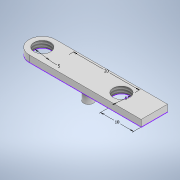
# Autodesk Inventor part: link
Saved by Autodesk Inventor 2021 (Build 250183000, 183)
## iProperties
Created: 2020-11-29
Part Number: link
Material: Generic
Document SubType Name: Modeling
Designer: awitc
Density: 1 g/cm^3
Appearance: Default
Author: awitc
Autodesk Inventor part; units mm, degrees
ref_plane "YZ Plane" through (0, 0, 0) normal (1, 0, 0) x (0, 1, 0)
ref_plane "XZ Plane" through (0, 0, 0) normal (0, 1, 0) x (-1, 0, 0)
ref_plane "XY Plane" through (0, 0, 0) normal (0, 0, 1) x (1, 0, 0)
sketch "Sketch1" plane through (0, 0, 0) normal (0, 1, 0) x (-1, 0, 0)
  line L0 (0, 4) -> (-20, 4)
  line L1 (-20, 4) -> (-20, -4)
  line L2 (-20, -4) -> (0, -4)
  circle A0 centre (-20, 0) radius 4
  circle A1 centre (-20, 0) radius 2.5
  line L3 (-20, -4) -> (-30, -4)
  line L4 (-30, -4) -> (-30, 4)
  line L5 (-30, 4) -> (-20, 4)
  line L6 (-20, 4) -> (-20, -4)
  circle A2 centre (4, 0) radius 4
  circle A3 centre (4, 0) radius 2.5
  line L7 (0, 4) -> (4, 4)
  line L8 (4, -4) -> (0, -4)
  point P0 (-20, -2.5)
  point P1 (-20, 2.5)
  dimension "d32" = 20
  dimension "d34" = 5
  dimension "d47" = 10
  dimension "d48" = 5
  constraints: 18 end point, 4 parallel, 3 centre point, 2 coincident, 2 horizontal, 2 perpendicular, 2 point on circle, 2 tangent, 1 midpoint, 3 other
  measures "d32" distance of L2.end L1.end
  measures "d34" diameter of A1
  measures "d47" distance of L4.end L5.end
  measures "d48" diameter of A3
extrude "Extrusion1" add sketch "Sketch1" along normal blind 2 contours L7 A2 L8 L2 A0 L0 | A0 L1 A1 | L1 A1 A0 | A0 L3 L4 L5 | A2
thread "Thread2" size "M5x0.8" class "6H" standard "ANSI Metric M Profile" full length
sketch "Sketch4" plane through (0, 0, 0) normal (0, -1, 0) x (1, 0, 0)
  circle A0 centre (10, 0) radius 1.5
  point P0 (0, 0)
  dimension "d46" = 3
  constraints: 1 centre point
  measures "d46" diameter of A0
extrude "Extrusion5" add sketch "Sketch4" along normal blind 5
thread "Thread3" size "M5x0.8" class "6H" standard "ANSI Metric M Profile" full length
body "Solid1"
